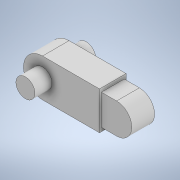
# Autodesk Inventor part: 03-2
Saved by Autodesk Inventor 2022 (Build 260153000, 153)
## iProperties
Created: 2021-09-11
Part Number: 03-2
Material: 일반
Document SubType Name: Modeling
Designer: 서울공업고등학교
Density: 1 g/cm^3
Appearance: 기본값
Author: 서울공업고등학교
Autodesk Inventor part; units mm, degrees
ref_plane "YZ Plane" through (0, 0, 0) normal (1, 0, 0) x (0, 1, 0)
ref_plane "XZ Plane" through (0, 0, 0) normal (0, 1, 0) x (-1, 0, 0)
ref_plane "XY Plane" through (0, 0, 0) normal (0, 0, 1) x (1, 0, 0)
sketch "스케치1" plane through (0, 0, 0) normal (0, 0, 1) x (1, 0, 0)
  line L0 (-10, 5) -> (10, 5)
  line L1 (10, 5) -> (10, -5)
  line L2 (10, -5) -> (-10, -5)
  line L3 (-10, -5) -> (-10, 5)
  line L4 (-10, 5) -> (10, -5) construction
  line L5 (10, 5) -> (-10, -5) construction
  line L6 (10, 4) -> (18, 4)
  line L7 (18, 4) -> (18, -4)
  line L8 (18, -4) -> (10, -4)
  line L9 (10, -4) -> (10, 4)
  circle A0 centre (-5, 0) radius 2.5
  point P0 (0, 0)
  point P1 (0, 0)
  point P2 (18, 0)
  dimension "d0" = 20
  dimension "d1" = 10
  dimension "d2" = 8
  dimension "d3" = 8
  dimension "d4" = 5
  dimension "d5" = 15
  dimension "d6" = 5
  constraints: 20 end point, 4 midpoint, 4 parallel, 2 horizontal, 2 perpendicular, 1 centre point, 1 horizontal alignment, 1 point on line
  measures "d0" distance of L1.end L2.end
  measures "d1" distance of L0.end L1.end
  measures "d2" distance of L6.start L6.end
  measures "d3" distance between parallel lines of L6 L8
  measures "d4" diameter of A0
  measures "d5" distance from line of L1 A0.centre
  measures "d6" distance from line of L0 A0.centre
extrude "돌출1" add sketch "스케치1" along normal mid plane 16 contours A0
extrude "돌출2" add sketch "스케치1" along normal mid plane 7 contours L0 L1 L2 L3
extrude "돌출3" add sketch "스케치1" along normal mid plane 6 contours L6 L7 L8 L1
fillet "모깎기1" radius 4 2 edges at (18, 4, 0) (18, -4, 0)
fillet "모깎기2" radius 5 2 edges at (-10, 5, 0) (-10, -5, 0)
